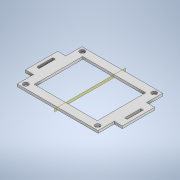
# Autodesk Inventor part: topBearingHolder
Saved by Autodesk Inventor 2020 (Build 240168000, 168)
## iProperties
Created: 2019-06-18
Part Number: topBearingHolder
Material: Generic
Document SubType Name: Modeling
Designer: Vivek Muskan
Density: 1 g/cm^3
Appearance: Default
Author: Vivek Muskan
Autodesk Inventor part; units mm, degrees
ref_plane "YZ Plane" through (0, 0, 0) normal (1, 0, 0) x (0, 1, 0)
sketch "Sketch1" plane through (0, 0, 0) normal (0, 1, 0) x (-1, 0, 0)
  circle A0 centre (0, 0) radius 8.5
  line L0 (19.5, 15) -> (-19.5, 15)
  line L1 (-19.5, 15) -> (-19.5, -15)
  line L2 (-19.5, -15) -> (19.5, -15)
  line L3 (19.5, -15) -> (19.5, 15)
  line L4 (19.5, 15) -> (-19.5, -15) construction
  line L5 (-19.5, 15) -> (19.5, -15) construction
  line L6 (25, 20) -> (-25, 20)
  line L7 (-25, 20) -> (-25, -20)
  line L8 (-25, -20) -> (25, -20)
  line L9 (25, -20) -> (25, 20)
  line L10 (25, 20) -> (-25, -20) construction
  line L11 (-25, 20) -> (25, -20) construction
  line L12 (-25, 0) -> (-30, 0)
  line L13 (-30, 0) -> (-30, -10)
  line L14 (-30, -10) -> (-25, -10)
  line L15 (-25, -10) -> (-25, 0)
  line L16 (-30, 0) -> (-25, 0)
  line L17 (-25, 0) -> (-25, 10)
  line L18 (-25, 10) -> (-30, 10)
  line L19 (-30, 10) -> (-30, 0)
  line L20 (-25, 10) -> (-25, 5)
  line L21 (-25, 5) -> (-26.5, 5)
  line L22 (-26.5, 5) -> (-28, 5)
  line L23 (-28, 5) -> (-28, -5)
  line L24 (-28, -5) -> (-26.5, -5)
  line L25 (-26.5, -5) -> (-26.5, 5)
  line L26 (0, 0) -> (0, -20)
  line L27 (30, 0) -> (30, -10)
  line L28 (30, -10) -> (25, -10)
  line L29 (25, 10) -> (30, 10)
  line L30 (30, 10) -> (30, 0)
  line L31 (26.5, 5) -> (28, 5)
  line L32 (28, 5) -> (28, -5)
  line L33 (28, -5) -> (26.5, -5)
  line L34 (26.5, -5) -> (26.5, 5)
  dimension "d0" = 17
  dimension "d1" = 39
  dimension "d2" = 30
  dimension "d3" = 50
  dimension "d4" = 40
  dimension "d5" = 5
  dimension "d6" = 10
  dimension "d7" = 5
  dimension "d8" = 10
  dimension "d9" = 5
  dimension "d10" = 1.5
  dimension "d11" = 1.5
  dimension "d12" = 10
  constraints: 70 end point, 10 parallel, 9 symmetric about line, 7 midpoint, 6 perpendicular, 5 horizontal, 1 centre point, 1 coincident
  measures "d0" diameter of A0
  measures "d1" distance of L2.end L1.end
  measures "d2" distance of L1.end L0.end
  measures "d3" distance of L8.end L7.end
  measures "d4" distance of L7.end L6.end
  measures "d5" distance of L14.end L13.end
  measures "d6" distance of L13.end L12.end
  measures "d7" distance of L18.end L17.end
  measures "d8" distance of L18.end L12.end
  measures "d9" distance of L17.end L20.end
  measures "d10" distance of L20.end L21.end
  measures "d11" distance of L24.end L23.end
  measures "d12" distance of L23.end L22.end
extrude "Extrusion1" add sketch "Sketch1" along normal blind 1.5 contours L8 L7 L6 L9 | L14 L13 L12 L23 L24 L25 L7 | L9 L29 L30 L27 L28 | L12 L25 L21 L7 | L21 L22 L23 L12 L19 L18 L7
sketch "Sketch2" plane through (0, 1.5, 0) normal (0, 1, 0) x (1, 0, 0)
  line L0 (19.5, -15) -> (-19.5, -15) projected
  line L1 (-19.5, -15) -> (-22.25, -15)
  line L2 (-22.25, -15) -> (-22.25, -17.5)
  line L3 (-25, -20) -> (25, -20) projected
  circle A0 centre (-22.25, -17.5) radius 1.5
  point P0 (0, 0)
  dimension "d15" = 2.75
  dimension "d16" = 2.5
  dimension "d17" = 3
  constraints: 4 end point, 1 centre point, 1 coincident, 1 horizontal, 1 perpendicular
  measures "d15" distance of L0.end L1.end
  measures "d16" distance of L1.end L2.end
  measures "d17" diameter of A0
extrude "Extrusion2" cut sketch "Sketch2" against normal blind 1.5
ref_plane "Work Plane1" through (0, 0, 10) normal (-1, 0, 0) x (0, 0, 1)
ref_plane "Work Plane2" through (25, 0, 0) normal (0, 0, -1) x (-1, 0, 0)
mirror "Mirror1" about plane through (0, 0, 10) normal (-1, 0, 0) of "Extrusion2"
mirror "Mirror2" about plane through (25, 0, 0) normal (0, 0, -1) of "Extrusion2", "Mirror1"
ref_plane "Work Plane3" through (0, 0, 10) normal (-1, 0, 0) x (0, 0, 1)
ref_plane "Work Plane4" through (0, 0, -10) normal (1, 0, 0) x (0, 0, -1)
ref_plane "Work Plane5" through (0, 0, -10) normal (1, 0, 0) x (0, 0, -1)
body "Solid1"
